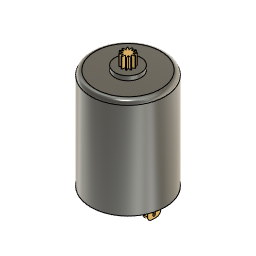
MG996R_Motor v4 (Autodesk Fusion 360 design; units mm, degrees)
Autodesk Fusion 360 part; units mm, degrees
note: some values were not read from the file. Chosen so that the rebuilt part matches the saved one: a direction. Set by a fixed rule: which sketch regions a step uses.
sketch "Sketch1" plane through (0, 0, 0) normal (0, 0, 1) x (1, 0, 0)
  circle A0 centre (0, 0) radius 8.5
  dimension "d1" = 17
  constraint coincident A0.centre origin
  measures "d1" diameter of A0
extrude "Extrude1" add sketch "Sketch1" along normal blind 23
sketch "Sketch2" plane through (0, 0, 23) normal (0, 0, 1) x (-1, 0, 0)
  circle A0 centre (0, 0) radius 8.5
  circle A1 centre (0, 0) radius 3
  dimension "d4" = 6
  constraint coincident A0.centre A1.centre
  measures "d4" diameter of A1
extrude "Extrude2" add sketch "Sketch2" along normal blind 1 contours A1
sketch "Sketch3" plane through (0, 0, 24) normal (0, 0, 1) x (-1, 0, 0)
  circle A0 centre (0, 0) radius 3
  circle A1 centre (0, 0) radius 1.5
  dimension "d7" = 3
  constraint concentric A0 A1
  measures "d7" diameter of A1
extrude "Extrude3" add sketch "Sketch3" along normal blind 2.5 contours A1
fillet "Fillet1" radius 1 1 edges at (-7.9248, -3.0737, 23)
sketch "Sketch4" plane through (0, 0, 0) normal (0, 0, -1) x (1, 0, 0)
  circle A0 centre (0, 0) radius 8.5
  line L0 (-5, 1.5) -> (-6, 1.5)
  line L1 (-6, 1.5) -> (-6, -1.5)
  line L2 (-6, -1.5) -> (-5, -1.5)
  line L3 (-5, -1.5) -> (-5, 1.5)
  line L4 (-5, 1.5) -> (-6, -1.5) construction
  line L5 (-6, 1.5) -> (-5, -1.5) construction
  line L6 (6, 1.5) -> (5, 1.5)
  line L7 (5, 1.5) -> (5, -1.5)
  line L8 (5, -1.5) -> (6, -1.5)
  line L9 (6, -1.5) -> (6, 1.5)
  line L10 (6, 1.5) -> (5, -1.5) construction
  line L11 (5, 1.5) -> (6, -1.5) construction
  point P0 (-5.5, 0)
  point P1 (5.5, 0)
  dimension "d12" = 1
  dimension "d13" = 1
  dimension "d14" = 3
  dimension "d15" = 3
  dimension "d16" = 5
  dimension "d17" = 5
  constraint horizontal L0
  constraint perpendicular L0 L1
  constraint parallel L0 L2
  constraint parallel L1 L3
  constraint coincident L4 P0
  constraint coincident L5 P0
  constraint horizontal L6
  constraint perpendicular L6 L7
  constraint parallel L6 L8
  constraint parallel L7 L9
  constraint coincident L10 P1
  constraint coincident L11 P1
  constraint horizontal A0.centre P0
  constraint horizontal A0.centre P1
  measures "d12" distance of L7 L9
  measures "d13" distance of L1 L3
  measures "d14" distance of L0.start L2.end
  measures "d15" distance of L6.end L7.end
  measures "d16" distance of A0.centre L3
  measures "d17" distance of A0.centre L7
extrude "Extrude4" add sketch "Sketch4" along normal blind 3.5 contours L0 L1 L2 L3 | L6 L7 L8 L9
sketch "Sketch5" plane through (-6, 0, 0) normal (-1, 0, 0) x (0, -1, 0)
  line L0 (1.5, 0) -> (-1.5, 0)
  line L1 (-1.5, 0) -> (-1.5, -3.5)
  line L2 (-1.5, -3.5) -> (1.5, -3.5)
  line L3 (1.5, -3.5) -> (1.5, 0)
  line L4 (0.25, -2.8) -> (0.25, -0.8)
  arc A0 (0.25, -0.8) -> (-0.25, -0.8) centre (0, -0.8) ccw
  line L5 (-0.25, -0.8) -> (-0.25, -2.8)
  arc A1 (-0.25, -2.8) -> (0.25, -2.8) centre (0, -2.8) ccw
  line L6 (0, -2.8) -> (0, -0.8) construction
  point P0 (0, -1.8)
  dimension "d20" = 2
  dimension "d21" = 0.5
  dimension "d22" = 0.7
  constraint tangent L4 A0
  constraint tangent A0 L5
  constraint parallel L4 L5
  constraint tangent L5 A1
  constraint tangent L4 A1
  constraint vertical L6
  constraint midpoint L6 P0
  constraint vertical origin A1.centre
  measures "d20" distance of L4.start L4.end
  measures "d21" distance of L4 L5
  measures "d22" distance of L2 A1.centre
extrude "Extrude5" cut sketch "Sketch5" against normal through all contours L4 A0 L5 A1
fillet "Fillet2" radius 1 4 edges at (-5.5, 1.5, -3.5) (-5.5, -1.5, -3.5) (5.5, 1.5, -3.5) (5.5, -1.5, -3.5)
sketch "Sketch6" plane through (0, 0, 26.5) normal (0, 0, 1) x (-1, 0, 0)
  circle A0 centre (0, 0) radius 1.5
  circle A1 centre (0, 0) radius 1.5
  line L0 (0.35, -1.4586) -> (0, -0.8524)
  line L1 (0, -0.8524) -> (-0.35, -1.4586)
  dimension "d26" = 0.7
  dimension "d27" = 0.7
  dimension "d28" = 0.7
  constraint concentric A0 A1
  constraint equal A0 A1
  constraint coincident A1 L0.start
  constraint coincident A1 L1.end
  constraint vertical A0.centre L0.end
  measures "d26" distance of L0.start L0.end
  measures "d27" distance of L0.end L1.end
  measures "d28" distance of L0.start L1.end
extrude "Extrude6" cut sketch "Sketch6" against normal blind 2.5 contours A0 A1 L0 L1 picked at (0.0587, -1.2807)
pattern_circular "C-Pattern1" count 11 over 360 about axis through (0, 0, 24) along (0, 0, 1) of "Extrude6"
